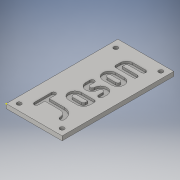
# Autodesk Inventor part: Jason_nameplate_lowered16
Saved by Autodesk Inventor 2016 (Build 200138000, 138)
## iProperties
Created: 2016-09-23
Part Number: Jason_nameplate_lowered16
Material: Generic
Document SubType Name: Modeling
Designer: jhaun
Density: 1 g/cm^3
Appearance: Default
Author: jhaun
Autodesk Inventor part; units mm, degrees
ref_plane "YZ Plane" through (0, 0, 0) normal (1, 0, 0) x (0, 1, 0)
ref_plane "XZ Plane" through (0, 0, 0) normal (0, 1, 0) x (-1, 0, 0)
ref_plane "XY Plane" through (0, 0, 0) normal (0, 0, 1) x (1, 0, 0)
sketch "Sketch1" plane through (0, 0, 0) normal (0, 1, 0) x (-1, 0, 0)
  line L0 (0, 0) -> (-82.55, 0)
  line L1 (-82.55, 0) -> (-82.55, -165.1)
  line L2 (-82.55, -165.1) -> (0, -165.1)
  line L3 (0, -165.1) -> (0, 0)
  circle A0 centre (-9.525, -9.525) radius 3.175
  circle A1 centre (-73.025, -9.525) radius 3.175
  circle A2 centre (-73.025, -155.575) radius 3.175
  circle A3 centre (-9.525, -152.4) radius 3.175
  constraints: 8 end point, 4 centre point, 2 parallel, 1 horizontal, 1 perpendicular
extrude "Extrusion1" add sketch "Sketch1" along normal blind 6.35
sketch "Sketch2" plane through (0, 6.35, 0) normal (0, 1, 0) x (1, 0, 0)
  arc A0 (19.05, 22.225) -> (25.4, 22.225) centre (22.225, 22.225) ccw
  line L0 (25.4, 22.225) -> (25.4, 31.75)
  line L1 (25.4, 31.75) -> (47.625, 31.75)
  arc A1 (57.15, 22.225) -> (47.625, 31.75) centre (47.625, 22.225) ccw
  arc A2 (57.15, 22.225) -> (63.5, 22.225) centre (60.325, 22.225) ccw
  arc A3 (63.5, 22.225) -> (47.625, 38.1) centre (47.625, 22.225) ccw
  line L2 (47.625, 38.1) -> (25.4, 38.1)
  line L3 (25.4, 38.1) -> (25.4, 47.625)
  arc A4 (25.4, 47.625) -> (19.05, 47.625) centre (22.225, 47.625) ccw
  line L4 (19.05, 47.625) -> (19.05, 22.225)
  arc A5 (41.275, 69.85) -> (41.275, 50.8) centre (41.275, 60.325) ccw
  arc A6 (41.275, 63.5) -> (41.275, 57.15) centre (41.275, 60.325) ccw
  arc A7 (31.75, 85.725) -> (50.8, 85.725) centre (41.275, 85.725) ccw
  arc A8 (38.1, 85.725) -> (44.45, 85.725) centre (41.275, 85.725) ccw
  arc A9 (57.15, 85.725) -> (50.8, 85.725) centre (53.975, 85.725) ccw
  arc A10 (63.5, 85.725) -> (44.45, 85.725) centre (53.975, 85.725) ccw
  line L5 (31.75, 85.725) -> (31.75, 92.075)
  arc A11 (38.1, 92.075) -> (31.75, 92.075) centre (34.925, 92.075) ccw
  arc A12 (57.15, 79.375) -> (63.5, 79.375) centre (60.325, 79.375) ccw
  line L6 (57.15, 85.725) -> (57.15, 79.375)
  line L7 (63.5, 79.375) -> (63.5, 85.725)
  line L8 (38.1, 85.725) -> (38.1, 92.075)
  arc A13 (53.975, 50.8) -> (63.5, 60.325) centre (53.975, 60.325) ccw
  arc A14 (53.975, 57.15) -> (57.15, 60.325) centre (53.975, 60.325) ccw
  line L9 (41.275, 50.8) -> (53.975, 50.8)
  line L10 (41.275, 57.15) -> (53.975, 57.15)
  line L11 (57.15, 60.325) -> (57.15, 63.5)
  line L12 (57.15, 63.5) -> (41.275, 63.5)
  arc A15 (41.275, 120.65) -> (41.275, 101.6) centre (41.275, 111.125) ccw
  arc A16 (41.275, 114.3) -> (41.275, 107.95) centre (41.275, 111.125) ccw
  arc A17 (53.975, 101.6) -> (53.975, 120.65) centre (53.975, 111.125) ccw
  arc A18 (53.975, 107.95) -> (53.975, 114.3) centre (53.975, 111.125) ccw
  line L13 (41.275, 101.6) -> (53.975, 101.6)
  line L14 (41.275, 107.95) -> (53.975, 107.95)
  line L15 (41.275, 114.3) -> (53.975, 114.3)
  line L16 (41.275, 120.65) -> (53.975, 120.65)
  arc A19 (60.325, 127) -> (60.325, 133.35) centre (60.325, 130.175) ccw
  line L17 (60.325, 127) -> (34.925, 127)
  arc A20 (31.75, 130.175) -> (34.925, 127) centre (34.925, 130.175) ccw
  line L18 (31.75, 130.175) -> (31.75, 136.525)
  line L19 (60.325, 133.35) -> (38.1, 133.35)
  line L20 (38.1, 133.35) -> (38.1, 136.525)
  arc A21 (41.275, 139.7) -> (38.1, 136.525) centre (41.275, 136.525) ccw
  arc A22 (41.275, 146.05) -> (31.75, 136.525) centre (41.275, 136.525) ccw
  line L21 (41.275, 139.7) -> (60.325, 139.7)
  arc A23 (60.325, 139.7) -> (60.325, 146.05) centre (60.325, 142.875) ccw
  line L22 (60.325, 146.05) -> (41.275, 146.05)
  line L23 (63.5, 60.325) -> (63.5, 66.675)
  arc A24 (63.5, 66.675) -> (60.325, 69.85) centre (60.325, 66.675) ccw
  line L24 (60.325, 69.85) -> (41.275, 69.85)
  point P0 (0, 0)
  constraints: 53 point on circle, 50 end point, 25 centre point, 10 horizontal, 10 vertical, 8 coincident, 3 perpendicular, 2 parallel, 2 point on line
sketch "Sketch3" plane through (0, 6.35, 0) normal (0, 1, 0) x (1, 0, 0)
  point P0 (0, 0)
extrude "Extrusion2" cut sketch "Sketch2" against normal blind 3.175
body "Solid1"
